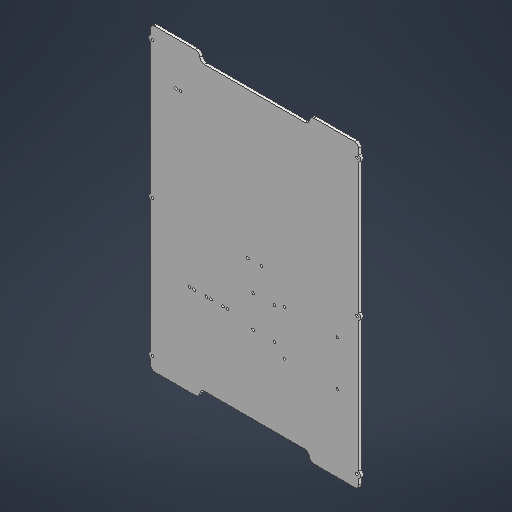
# Autodesk Inventor part: Control layer
Saved by Autodesk Inventor 2026.1 (Build 301233000, 233)
## iProperties
Created: 2026-03-06
Part Number: Control layer
Material: Generic
Document SubType Name: Modeling
Designer: momen
Density: 1 g/cm^3
Appearance: Default
Author: momen
Autodesk Inventor part; units mm, degrees
ref_plane "YZ Plane" through (0, 0, 0) normal (1, 0, 0) x (0, 1, 0)
ref_plane "XZ Plane" through (0, 0, 0) normal (0, 1, 0) x (-1, 0, 0)
ref_plane "XY Plane" through (0, 0, 0) normal (0, 0, 1) x (1, 0, 0)
sketch "Sketch1" plane through (0, 0, 0) normal (0, 0, 1) x (1, 0, 0)
  line L0 (-114, -164) -> (114, -164)
  line L1 (114, 164) -> (-114, 164)
  line L2 (-114, -164) -> (114, 164) construction
  line L3 (114, -164) -> (-114, 164) construction
  line L4 (-112, -150) -> (112, -150)
  line L5 (112, -150) -> (112, 150)
  line L6 (112, 150) -> (-112, 150)
  line L7 (-112, 150) -> (-112, -150)
  line L8 (-112, -150) -> (112, 150) construction
  line L9 (112, -150) -> (-112, 150) construction
  circle A0 centre (112, 150) radius 1.5
  arc A1 (114, 146.5359) -> (114, 153.4641) centre (112, 150) ccw
  line L10 (114, 153.4641) -> (114, 164)
  line L11 (0, -56.7016) -> (0, 56.7016)
  line L12 (-37.0034, 0) -> (37.0034, 0)
  circle A2 centre (-112, 150) radius 1.5
  arc A3 (-114, 153.4641) -> (-114, 146.5359) centre (-112, 150) ccw
  circle A4 centre (112, -150) radius 1.5
  arc A5 (114, -153.4641) -> (114, -146.5359) centre (112, -150) ccw
  arc A6 (-114, -146.5359) -> (-114, -153.4641) centre (-112, -150) ccw
  circle A7 centre (-112, -150) radius 1.5
  line L13 (-114, 164) -> (-114, 153.4641)
  line L14 (114, -164) -> (114, -153.4641)
  line L15 (-114, -153.4641) -> (-114, -164)
  circle A8 centre (112, 0) radius 1.5
  arc A9 (114, -3.4641) -> (114, 3.4641) centre (112, 0) ccw
  line L16 (114, -146.5359) -> (114, -3.4641)
  line L17 (114, 3.4641) -> (114, 146.5359)
  circle A10 centre (-112, 0) radius 1.5
  arc A11 (-114, 3.4641) -> (-114, -3.4641) centre (-112, 0) ccw
  line L18 (-114, 146.5359) -> (-114, 3.4641)
  line L19 (-114, -3.4641) -> (-114, -146.5359)
  line L20 (-60, 164) -> (60, 164)
  line L21 (60, 164) -> (-60, 164)
  line L22 (-60, 164) -> (-60, 155)
  line L23 (-60, 155) -> (60, 155)
  line L24 (60, 155) -> (60, 164)
  line L25 (-60, -164) -> (-60, -155)
  line L26 (-60, -155) -> (60, -155)
  line L27 (60, -155) -> (60, -164)
  point P0 (0, 0)
  point P1 (0, 164)
  dimension "d0" = 228
  dimension "d1" = 328
  dimension "d2" = 224
  dimension "d3" = 300
  dimension "d4" = 3
  dimension "d10" = 3
  dimension "d11" = 8
  dimension "d12" = 120
  dimension "d13" = 120
  dimension "d14" = 9
  constraints: 56 end point, 21 parallel, 20 symmetric about line, 12 centre point, 12 point on circle, 9 midpoint, 7 coincident, 6 perpendicular, 4 horizontal, 1 point on line, 1 vertical, 8 other
  measures "d0" distance of L1.end L1.start
  measures "d1" distance of L1.start L0.end
  measures "d2" distance of L6.end L5.end
  measures "d3" distance of L5.end L4.end
  measures "d4" diameter of A0
  measures "d10" diameter of A8
  measures "d11" diameter of A9
  measures "d12" distance of L20.start L20.end
  measures "d13" distance of L23.end L22.end
  measures "d14" distance of L22.end L21.end
extrude "Extrusion1" add sketch "Sketch1" along normal blind 3 contours L15 A6 L19 A11 L18 A3 L13 L1 L22 L23 L24 L10 A1 L17 A9 L16 A5 L14 L0 L27 L26 L25 | A7 L7 A10 A2 L6 A0 L5 A8 A4 L4
fillet "Fillet1" radius 4.1 4 edges at (114, 164, 1.5) (114, -164, 1.5) (-114, 164, 1.5) (-114, -164, 1.5)
fillet "Fillet2" radius 5 8 edges at (-60, 164, 1.5) (60, 164, 1.5) (60, 155, 1.5) (-60, 155, 1.5) (-60, -164, 1.5) (-60, -155, 1.5) (60, -155, 1.5) (60, -164, 1.5)
sketch "Sketch3" plane through (0, 0, 3) normal (0, 0, 1) x (1, 0, 0)
  circle A0 centre (-66.131, -64.28) radius 1.5 projected
  circle A1 centre (-71.131, -64.28) radius 1.5 projected
  circle A2 centre (-52.931, -64.28) radius 1.5 projected
  circle A3 centre (-47.931, -64.28) radius 1.5 projected
  circle A4 centre (-34.731, -64.28) radius 1.5 projected
  circle A5 centre (-29.731, -64.28) radius 1.5 projected
  circle A6 centre (-1.75, -35.23) radius 1.45 projected
  circle A7 centre (21.55, -35.23) radius 1.45 projected
  circle A8 centre (-1.75, -70.23) radius 1.45 projected
  circle A9 centre (21.55, -70.23) radius 1.45 projected
  circle A10 centre (32.5, -80.28) radius 1.35 projected
  circle A11 centre (32.5, -31.28) radius 1.35 projected
  circle A12 centre (90.5, -80.28) radius 1.35 projected
  circle A13 centre (90.5, -31.28) radius 1.35 projected
  circle A14 centre (-86.131, 116.72) radius 1.5 projected
  circle A15 centre (-81.131, 116.72) radius 1.5 projected
  circle A16 centre (-7.4766, -5.121) radius 1.5084 projected
  circle A17 centre (7.5843, -5.1439) radius 1.4324 projected
  point P0 (0, 0)
extrude "Extrusion3" cut sketch "Sketch3" against normal blind 3
body "Solid1"
